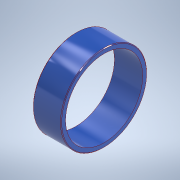
# Autodesk Inventor part: Промежуточное колесо резина
Saved by Autodesk Inventor 2021 (Build 250183000, 183)
## iProperties
Created: 2023-03-30
Part Number: Промежуточное колесо резина
Material: Резина
Document SubType Name: Modeling
Designer: gdevc
Density: 0.93 g/cm^3
Appearance: Светло-красный
Author: gdevc
Autodesk Inventor part; units mm, degrees
ref_plane "YZ Plane" through (0, 0, 0) normal (1, 0, 0) x (0, 1, 0)
ref_plane "XZ Plane" through (0, 0, 0) normal (0, 1, 0) x (-1, 0, 0)
ref_plane "XY Plane" through (0, 0, 0) normal (0, 0, 1) x (1, 0, 0)
sketch "Эскиз1" plane through (0, 0, 0) normal (0, 0, 1) x (1, 0, 0)
  line L0 (0, 33.5) -> (22, 33.5)
  line L1 (22, 33.5) -> (22, 0)
  line L2 (22, 0) -> (0, 0)
  line L3 (0, 0) -> (0, 33.5)
  line L4 (-4.4, 0) -> (26.4, 0) projected
  dimension "d0" = 33.5
  dimension "d1" = 22
  constraints: 8 end point, 2 parallel, 2 point on line, 1 horizontal, 1 perpendicular
  measures "d0" distance between parallel lines of L2 L0
  measures "d1" distance of L1.end L2.end
revolve "Вращение1" add sketch "Эскиз1" angle 360 about axis through (-10, 0, 0) along (1, 0, 0)
sketch "Эскиз3" plane through (22, 0, 0) normal (1, 0, 0) x (0, 0, -1)
  circle A0 centre (0, 0) radius 30
  dimension "d3" = 60
  constraints: 1 centre point, 1 coincident
  measures "d3" diameter of A0
extrude "Выдавливание1" cut sketch "Эскиз3" against normal through all
chamfer "Фаска1" distance 0.5 angle 45 2 edges at (22, -33.5, 0) (0, -33.5, 0)
